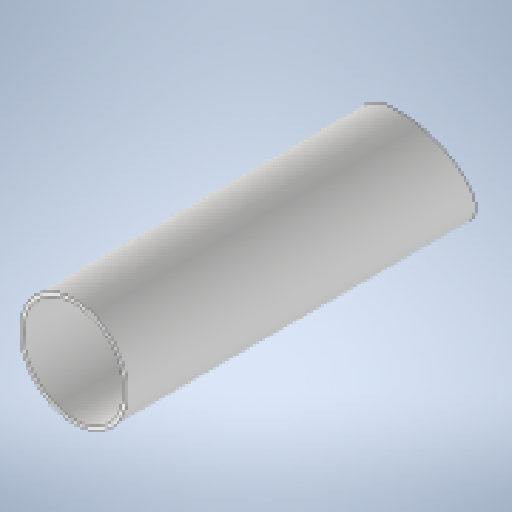
# Autodesk Inventor part: МОО 065 ракета труба 5
Saved by Autodesk Inventor 2025 (Build 290162010, 162A)
## iProperties
Created: 2024-05-24
Part Number: МОО 065 ракета труба 5
Material: Generic
Document SubType Name: Modeling
Designer: admin
Density: 1 g/cm^3
Appearance: Default
Author: admin
Autodesk Inventor part; units mm, degrees
ref_plane "YZ Plane" through (0, 0, 0) normal (1, 0, 0) x (0, 1, 0)
ref_plane "XZ Plane" through (0, 0, 0) normal (0, 1, 0) x (-1, 0, 0)
ref_plane "XY Plane" through (0, 0, 0) normal (0, 0, 1) x (1, 0, 0)
sketch "Sketch1" plane through (0, 0, 0) normal (0, 0, 1) x (1, 0, 0)
  circle A0 centre (0, 0) radius 44.5
  circle A1 centre (0, 0) radius 41.5
  dimension "d0" = 89
  dimension "d1" = 3
  constraints: 2 centre point, 1 coincident
  measures "d0" diameter of A0
  measures "d1" radial gap between concentric circles of A0 A1
extrude "Extrusion1" add sketch "Sketch1" along normal blind 300
sketch "Sketch2" plane through (0, 0, 0) normal (1, 0, 0) x (0, 1, 0)
  line L0 (44.5, 300) -> (-44.5, 300) projected
  line L1 (44.5, 0) -> (-44.5, 0) projected
  line L2 (-44.5, 0) -> (44.5, 32.3934)
  line L3 (44.5, 32.3934) -> (44.5, 0)
  line L4 (44.5, 0) -> (44.5, 300) projected
  point P0 (0, 0)
  dimension "d4" = 20
  constraints: 4 end point, 1 collinear
  measures "d4" angle of L2 L1
extrude "Extrusion2" cut sketch "Sketch2" along normal mid plane 300
body "Solid1"
